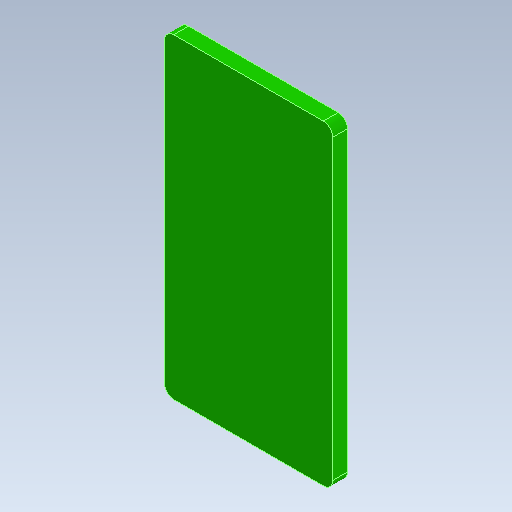
# Autodesk Inventor part: USB_MAIN_EXTENSION_PCB
Saved by Autodesk Inventor 2021 (Build 250183000, 183)
## iProperties
Created: 2020-06-15
Part Number: USB_MAIN_EXTENSION_PCB
Material: Generic
Document SubType Name: Modeling
Designer: Viktor Lindström
Density: 1 g/cm^3
Appearance: Default
Author: Viktor Lindström
Autodesk Inventor part; units mm, degrees
ref_plane "YZ Plane" through (0, 0, 0) normal (1, 0, 0) x (0, 1, 0)
ref_plane "XZ Plane" through (0, 0, 0) normal (0, 1, 0) x (-1, 0, 0)
ref_plane "XY Plane" through (0, 0, 0) normal (0, 0, 1) x (1, 0, 0)
sketch "Sketch1" plane through (0, 0, 0) normal (0, 0, 1) x (1, 0, 0)
  line L0 (-9, -16.9) -> (9, -16.9)
  line L1 (9, -16.9) -> (9, 16.9)
  line L2 (9, 16.9) -> (-9, 16.9)
  line L3 (-9, 16.9) -> (-9, -16.9)
  line L4 (-9, -16.9) -> (9, 16.9) construction
  line L5 (9, -16.9) -> (-9, 16.9) construction
  point P0 (0, 0)
  dimension "d0" = 18
  dimension "d1" = 33.8
  constraints: 12 end point, 2 midpoint, 2 parallel, 1 horizontal, 1 perpendicular
  measures "d0" distance of L1.end L2.end
  measures "d1" distance of L2.end L0.start
extrude "Extrusion1" add sketch "Sketch1" along normal mid plane 1.6
fillet "Fillet1" radius 1 4 edges at (-9, -16.9, 0) (9, -16.9, 0) (9, 16.9, 0) (-9, 16.9, 0)
sketch "USB_MAIN_EXTENSION_PCB_OUTLINE" plane through (0, 0, 0.8) normal (0, 0, 1) x (1, 0, 0)
  arc A0 (-8, 16.9) -> (-9, 15.9) centre (-8, 15.9) ccw projected
  line L0 (-9, 15.9) -> (-9, -15.9) projected
  arc A1 (-9, -15.9) -> (-8, -16.9) centre (-8, -15.9) ccw projected
  line L1 (-8, -16.9) -> (8, -16.9) projected
  arc A2 (8, -16.9) -> (9, -15.9) centre (8, -15.9) ccw projected
  line L2 (9, -15.9) -> (9, 15.9) projected
  arc A3 (9, 15.9) -> (8, 16.9) centre (8, 15.9) ccw projected
  line L3 (8, 16.9) -> (-8, 16.9) projected
  line L4 (7, 13.9) -> (7, 8.515)
  line L5 (7, 8.485) -> (7, 3.1)
  line L6 (7, -3.1) -> (7, -8.485)
  line L7 (7, -8.515) -> (7, -13.9)
  line L8 (3.15, -14.5) -> (4.75, -14.5)
  line L9 (4.75, -14.2) -> (3.15, -14.2)
  line L10 (4.95, -14.5) -> (4.95, -14.2)
  line L11 (2.95, -14.2) -> (2.95, -14.5)
  line L12 (4.75, -2.5) -> (3.15, -2.5)
  line L13 (3.15, -2.8) -> (4.75, -2.8)
  line L14 (4.95, -2.8) -> (4.95, -2.5)
  line L15 (2.95, -2.5) -> (2.95, -2.8)
  line L16 (4.75, 2.8) -> (3.15, 2.8)
  line L17 (3.15, 2.5) -> (4.75, 2.5)
  line L18 (4.95, 2.5) -> (4.95, 2.8)
  line L19 (2.95, 2.8) -> (2.95, 2.5)
  line L20 (4.75, 14.5) -> (3.15, 14.5)
  line L21 (3.15, 14.2) -> (4.75, 14.2)
  line L22 (4.95, 14.2) -> (4.95, 14.5)
  line L23 (2.95, 14.5) -> (2.95, 14.2)
  line L24 (2.2526, 12.7) -> (1.15, 12.7)
  line L25 (1.05, 12.4) -> (1.05, 12.6)
  line L26 (1.15, 4.3) -> (2.2526, 4.3)
  line L27 (1.05, 4.4) -> (1.05, 4.6)
  line L28 (2.2526, -4.3) -> (1.15, -4.3)
  line L29 (1.05, -4.6) -> (1.05, -4.4)
  line L30 (1.15, -12.7) -> (2.2526, -12.7)
  line L31 (1.05, -12.6) -> (1.05, -12.4)
  circle A4 centre (3.95, -2.65) radius 1
  circle A5 centre (3.95, -14.35) radius 1
  circle A6 centre (3.95, 2.65) radius 1
  circle A7 centre (3.95, 14.35) radius 1
  line L32 (-6.755, -9.254) -> (-6.755, -8.746)
  line L33 (-6.247, -8.746) -> (-6.755, -8.746)
  line L34 (-6.247, -9.254) -> (-6.247, -8.746)
  line L35 (-6.755, -9.254) -> (-6.247, -9.254)
  line L36 (-4.755, 8.746) -> (-4.755, 9.254)
  line L37 (-4.247, 8.746) -> (-4.755, 8.746)
  line L38 (-4.247, 8.746) -> (-4.247, 9.254)
  line L39 (-4.247, 9.254) -> (-4.755, 9.254)
  circle A8 centre (-4.501, 9) radius 0.254
  circle A9 centre (-6.501, -9) radius 0.254
  point P0 (0, 0)
  constraints: 72 end point, 16 vertical, 12 horizontal, 6 centre point, 3 tangent, 72 other
body "Solid1"
